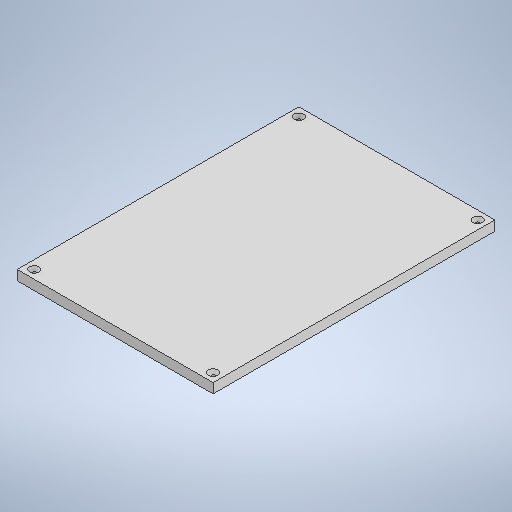
# Autodesk Inventor part: Honigschleuder_Steuerung_Deckel
Saved by Autodesk Inventor 2025 (Build 290162010, 162A)
## iProperties
Created: 2025-12-05
Part Number: Honigschleuder_Steuerung_Deckel
Material: Generisch
Document SubType Name: Modeling
Designer: max-h
Density: 1 g/cm^3
Appearance: Vorgabe
Author: max-h
Autodesk Inventor part; units mm, degrees
ref_plane "YZ Plane" through (0, 0, 0) normal (1, 0, 0) x (0, 1, 0)
ref_plane "XZ Plane" through (0, 0, 0) normal (0, 1, 0) x (-1, 0, 0)
ref_plane "XY Plane" through (0, 0, 0) normal (0, 0, 1) x (1, 0, 0)
sketch "Skizze1" plane through (0, 0, 0) normal (0, 1, 0) x (-1, 0, 0)
  line L0 (0, 0) -> (-80, 0)
  line L1 (-80, 0) -> (-80, -115)
  line L2 (-80, -115) -> (0, -115)
  line L3 (0, -115) -> (0, 0)
  line L4 (-3.5, -3.5) -> (-76.5, -3.5) construction
  line L5 (-76.5, -3.5) -> (-76.5, -111.5) construction
  line L6 (-76.5, -111.5) -> (-3.5, -111.5) construction
  line L7 (-3.5, -111.5) -> (-3.5, -3.5) construction
  circle A0 centre (-3.5, -3.5) radius 0.7
  circle A1 centre (-3.5, -111.5) radius 0.7
  circle A2 centre (-76.5, -111.5) radius 0.7
  circle A3 centre (-76.5, -3.5) radius 0.7
  dimension "d0" = 115
  dimension "d1" = 80
  dimension "d2" = 3.5
  dimension "d3" = 1.4
  constraints: 16 end point, 5 coincident, 4 centre point, 4 parallel, 3 equal radius, 2 perpendicular, 1 horizontal, 3 other
  measures "d0" distance of L2.end L0.start
  measures "d1" distance of L0.start L0.end
  measures "d2" distance between parallel lines of L3 L7
  measures "d3" diameter of A0
extrude "Extrusion1" add sketch "Skizze1" along normal blind 4
chamfer "Fasen1" distance 1.2 angle 45 4 edges at (4.2, 4, -3.5) (4.2, 4, -111.5) (77.2, 4, -111.5) (77.2, 4, -3.5)
sketch "Skizze2" plane through (0, 0, 0) normal (0, -1, 0) x (1, 0, 0)
  line L0 (29, -90) -> (46.5, -90) construction
  line L1 (46.5, -90) -> (46.5, -20) construction
  line L2 (46.5, -20) -> (29, -20) construction
  line L3 (29, -20) -> (29, -90) construction
  line L4 (0, -115) -> (0, 0) construction
  line L5 (47.5, -90) -> (65, -90) construction
  line L6 (65, -90) -> (65, -20) construction
  line L7 (65, -20) -> (47.5, -20) construction
  line L8 (47.5, -20) -> (47.5, -90) construction
  line L9 (80, -115) -> (0, -115) construction
  circle A0 centre (31, -88) radius 2.5
  arc A1 (44.5, -85.5) -> (44.5, -90.5) centre (44.5, -88) ccw
  circle A2 centre (63, -88) radius 2.5
  circle A3 centre (31, -22) radius 2.5
  arc A4 (44.5, -19.5) -> (44.5, -24.5) centre (44.5, -22) ccw
  arc A5 (49.5, -24.5) -> (49.5, -19.5) centre (49.5, -22) ccw
  circle A6 centre (63, -22) radius 2.5
  line L10 (31, -88) -> (44.5, -88) construction
  line L11 (44.5, -88) -> (44.5, -22) construction
  line L12 (44.5, -22) -> (31, -22) construction
  line L13 (31, -22) -> (31, -88) construction
  line L14 (49.5, -88) -> (63, -88) construction
  line L15 (63, -88) -> (63, -22) construction
  line L16 (63, -22) -> (49.5, -22) construction
  line L17 (49.5, -22) -> (49.5, -88) construction
  line L18 (44.5, -90.5) -> (49.5, -90.5)
  line L19 (44.5, -85.5) -> (49.5, -85.5)
  line L20 (44.5, -24.5) -> (49.5, -24.5)
  line L21 (44.5, -19.5) -> (49.5, -19.5)
  arc A7 (49.5, -90.5) -> (49.5, -85.5) centre (49.5, -88) ccw
  dimension "d9" = 29
  dimension "d10" = 17.5
  dimension "d11" = 70
  dimension "d12" = 25
  dimension "d13" = 1
  dimension "d14" = 2
  dimension "d15" = 2
  dimension "d16" = 5
  constraints: 40 end point, 10 parallel, 8 centre point, 8 coincident, 8 point on circle, 6 equal radius, 5 point on line, 4 perpendicular, 3 equal length, 2 horizontal, 1 collinear, 1 tangent, 6 other
  measures "d9" distance between parallel lines of L4 L3
  measures "d10" distance of L0.start L0.end
  measures "d11" distance of L0.end L1.end
  measures "d12" distance between parallel lines of L9 L0
  measures "d13" distance between parallel lines of L1 L8
  measures "d14" distance between parallel lines of L3 L13
  measures "d15" distance between parallel lines of L8 L17
  measures "d16" diameter of A0
extrude "Extrusion2" add sketch "Skizze2" along normal blind 4
sketch "Skizze3" plane through (31, -4, -22) normal (0, -1, 0) x (1, 0, 0)
  circle A0 centre (0, 0) radius 0.7
  arc A1 (13.5, 2.5) -> (13.5, -2.5) centre (13.5, 0) ccw projected
  circle A2 centre (13.5, 0) radius 0.7
  circle A3 centre (32, 0) radius 2.5 projected
  circle A4 centre (32, 0) radius 0.7
  arc A5 (18.5, -2.5) -> (18.5, 2.5) centre (18.5, 0) ccw projected
  circle A6 centre (18.5, 0) radius 0.7
  circle A7 centre (0, -66) radius 0.7
  arc A8 (13.5, -63.5) -> (13.5, -68.5) centre (13.5, -66) ccw projected
  circle A9 centre (13.5, -66) radius 0.7
  arc A10 (18.5, -68.5) -> (18.5, -63.5) centre (18.5, -66) ccw projected
  circle A11 centre (18.5, -66) radius 0.7
  circle A12 centre (32, -66) radius 0.7
  circle A13 centre (0, 0) radius 2.5 projected
  circle A14 centre (0, -66) radius 2.5 projected
  circle A15 centre (32, -66) radius 2.5 projected
  point P0 (-31, 22)
  dimension "d19" = 1.4
  constraints: 8 centre point, 8 coincident, 7 equal radius
  measures "d19" diameter of A0
extrude "Extrusion3" cut sketch "Skizze3" against normal blind 5 contours A0 | A2 | A4 | A6 | A7 | A9 | A11 | A12
